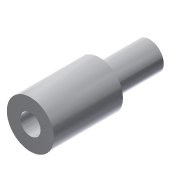
# Autodesk Inventor part: PP-04
Saved by Autodesk Inventor 2022 (Build 260148000, 148)
## iProperties
Created: 2008-09-23
Part Number: PP-04
Document SubType Name: Modeling
Designer: Mark Flayler
Mass: 0.034267 g
Surface Area: 0.976564 cm^2
Volume: 0.0323274 cm^3
Density: 1.06 g/cm^3
Material: ABS Plastic
Description: COUPLING
Appearance: Smooth - White
Author: Mark Flayler
Autodesk Inventor part; units mm, degrees
ref_plane "YZ Plane" through (0, 0, 0) normal (1, 0, 0) x (0, 1, 0)
ref_plane "XZ Plane" through (0, 0, 0) normal (0, 1, 0) x (-1, 0, 0)
ref_plane "XY Plane" through (0, 0, 0) normal (0, 0, 1) x (1, 0, 0)
sketch "Sketch1" plane through (0, 0, 0) normal (0, 0, 1) x (1, 0, 0)
  line L0 (0, 0) -> (0, 7.6)
  line L1 (0.65, 0) -> (1.5, 0)
  line L2 (1.5, 0) -> (1.5, 4.4)
  line L3 (1.5, 4.4) -> (0.9, 4.4)
  line L4 (0.9, 4.4) -> (0.9, 7.6)
  line L5 (0.9, 7.6) -> (0.5, 7.6)
  line L6 (0.5, 7.6) -> (0.5, 1.75)
  line L7 (0.5, 1.75) -> (0.65, 1.75)
  line L8 (0.65, 1.75) -> (0.65, 0)
  dimension "d0" = 1
  dimension "d1" = 1.3
  dimension "d2" = 7.6
  dimension "d3" = 4.4
  dimension "d4" = 1.75
  dimension "d5" = 3
  dimension "d6" = 1.8
  constraints: 18 end point, 4 parallel, 4 perpendicular, 2 horizontal alignment, 1 vertical
  measures "d0" diameter of L6 L0
  measures "d1" diameter of L8 L0
  measures "d2" distance between parallel lines of L1 L5
  measures "d3" distance between parallel lines of L3 L1
  measures "d4" distance between parallel lines of L1 L7
  measures "d5" diameter of L2 L0
  measures "d6" diameter of L4 L0
revolve "Revolution1" add sketch "Sketch1" angle 360 about axis through (0, 0, 0) along (0, 1, 0)
body "Solid1"
